Autodesk Inventor part; units mm, degrees
(part 2 of 2)
sketch "Sketch9" plane through (0, 0, 15) normal (0, 0, 1) x (1, 0, 0)
  circle A0 centre (-80.5289, 0.8706) radius 14
  circle A1 centre (-42.1773, 17.6229) radius 1.6
  circle A2 centre (-23.1773, 17.6229) radius 1.6
  circle A3 centre (-48.9273, -13.1271) radius 1.6
  circle A4 centre (-16.4273, -13.1271) radius 1.6
  circle A5 centre (-80.5289, 0.8706) radius 14
  circle A6 centre (-42.1773, 17.6229) radius 1.6
  circle A7 centre (-23.1773, 17.6229) radius 1.6
  circle A8 centre (-48.9273, -13.1271) radius 1.6
  circle A9 centre (-16.4273, -13.1271) radius 1.6
  arc A10 (-87.8309, -10.1732) -> (-72.9926, -10.0147) centre (-80.5289, 0.8706) ccw projected
  point P0 (0, 0)
  dimension "d202" = -16.752
  dimension "d203" = 19
  dimension "d204" = 32.5
  dimension "d205" = -30.75
  dimension "d206" = 6.75
  dimension "d207" = 38.352
  constraints: 10 centre point, 6 coincident, 5 concentric
  measures "d203" distance of A2.centre A1.centre
  measures "d204" distance of A4.centre A3.centre
  measures "d205" vertical distance of A1.centre A3.centre
  measures "d206" horizontal distance of A3.centre A1.centre
extrude "Extrusion7" cut sketch "Sketch9" against normal blind 10 contours A1 | A2 | A3 | A4
body "Solid3"
